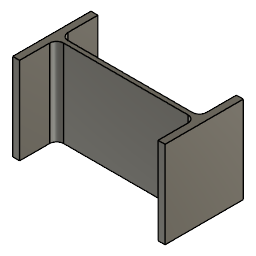
H-175×90×5×8 (Autodesk Fusion 360 design; units mm, degrees)
Autodesk Fusion 360 part; units mm, degrees
sketch "スケッチ1" plane through (0, 0, 0) normal (0, 0, 1) x (1, 0, 0)
  line L0 (159, 2.5) -> (16, 2.5)
  line L1 (16, -2.5) -> (159, -2.5)
  line L2 (0, 45) -> (0, -45)
  line L3 (8, -45) -> (8, -10.5)
  line L4 (0, -45) -> (8, -45)
  line L5 (8, 10.5) -> (8, 45)
  line L6 (8, 45) -> (0, 45)
  line L7 (175, -45) -> (175, 45)
  line L8 (167, -10.5) -> (167, -45)
  line L9 (167, -45) -> (175, -45)
  line L10 (167, 45) -> (167, 10.5)
  line L11 (175, 45) -> (167, 45)
  arc A0 (16, -2.5) -> (8, -10.5) centre (16, -10.5) ccw
  arc A1 (8, 10.5) -> (16, 2.5) centre (16, 10.5) ccw
  arc A2 (159, 2.5) -> (167, 10.5) centre (159, 10.5) ccw
  arc A3 (167, -10.5) -> (159, -2.5) centre (159, -10.5) ccw
extrude "押し出し1" add sketch "スケッチ1" along normal blind 100
